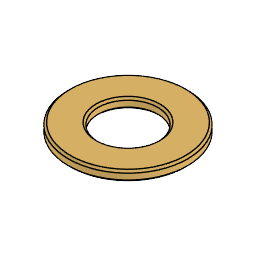
M3 Shim 0.5mm x 6mm (Autodesk Fusion 360 design; units mm, degrees)
Autodesk Fusion 360 part; units mm, degrees
sketch "Sketch1" plane through (0, 0, 0) normal (0, 0, 1) x (1, 0, 0)
  circle A0 centre (0, 0) radius 1.5
  circle A1 centre (0, 0) radius 3
  dimension "d1" = 3
  dimension "d2" = 6
  constraint coincident A0.centre A1.centre
  constraint concentric A0 A1
  measures "d1" diameter of A0
  measures "d2" diameter of A1
extrude "Extrude1" add sketch "Sketch1" along normal mid plane 0.5
chamfer "Chamfer1" distance 0.1 angle 45 4 edges at (-1.3985, 0.5424, 0.25) (-2.797, -1.0848, 0.25) (-2.797, 1.0848, -0.25) (-1.3985, -0.5424, -0.25)
